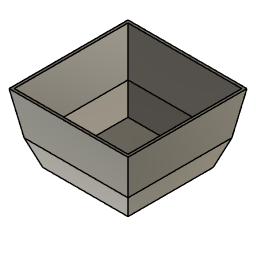
10411박서연_사각통_ (Autodesk Fusion 360 design; units mm, degrees)
Autodesk Fusion 360 part; units mm, degrees
sketch "스케치1" plane through (0, 0, 0) normal (0, 0, 1) x (1, 0, 0) in component "Component'"
  line L0 (-50, 50) -> (50, 50)
  line L1 (50, 50) -> (50, -50)
  line L2 (50, -50) -> (-50, -50)
  line L3 (-50, -50) -> (-50, 50)
  line L4 (-150, -30) -> (-65.8539, -30)
  line L5 (-65.8539, -30) -> (-94.1954, 36.1303)
  line L6 (-94.1954, 36.1303) -> (-70, 20)
  line L7 (-70, 20) -> (-80, 50)
  constraint horizontal L0
  constraint vertical L1
  constraint horizontal L2
  constraint vertical L3
  constraint horizontal L4
extrude "돌출1" add sketch "스케치1" along normal blind 30 draft 20 in component "Component'"
extrude "돌출2" add 1 faces at (-20.3064, 20.3064, 30) along direction (0, 0, 1) blind 50 draft 10 in component "Component'"
shell "쉘1" thickness 3 removed faces 1 at (-23.2452, 23.2452, 80) in component "Component'"
component "Component'" placed x (1, 0, 0) y (0, 1, 0) z (0, 0, 1) at (0, 0, 0)
